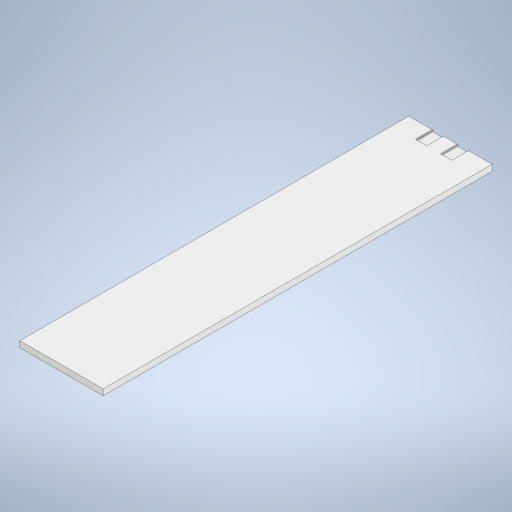
# Autodesk Inventor part: Resistance_chauffante_ceramique
Saved by Autodesk Inventor 2024 (Build 280153000, 153)
## iProperties
Created: 2024-08-30
Part Number: Resistance_chauffante_ceramique
Material: Générique
Document SubType Name: Modeling
Designer: malam
Density: 1 g/cm^3
Appearance: Par défaut
Author: malam
Autodesk Inventor part; units mm, degrees
ref_plane "YZ Plane" through (0, 0, 0) normal (1, 0, 0) x (0, 1, 0)
ref_plane "XZ Plane" through (0, 0, 0) normal (0, 1, 0) x (-1, 0, 0)
ref_plane "XY Plane" through (0, 0, 0) normal (0, 0, 1) x (1, 0, 0)
sketch "Esquisse1" plane through (0, 0, 0) normal (0, 1, 0) x (-1, 0, 0)
  line L0 (-7.5, 35) -> (7.5, 35)
  line L1 (7.5, 35) -> (7.5, -35)
  line L2 (7.5, -35) -> (-7.5, -35)
  line L3 (-7.5, -35) -> (-7.5, 35)
  line L4 (-7.5, 35) -> (7.5, -35) construction
  line L5 (7.5, 35) -> (-7.5, -35) construction
  point P0 (0, 0)
  dimension "d0" = 15
  dimension "d1" = 70
  constraints: 12 end point, 2 midpoint, 2 parallel, 1 horizontal, 1 perpendicular
  measures "d0" distance of L1.end L2.end
  measures "d1" distance of L0.end L1.end
extrude "Extrusion1" add sketch "Esquisse1" along normal blind 1.1
sketch "Esquisse2" plane through (0, 1.1, 0) normal (0, 1, 0) x (1, 0, 0)
  line L0 (7.5, 35) -> (-7.5, 35) projected
  line L1 (1.25, 35) -> (3.25, 35)
  line L2 (3.25, 35) -> (3.25, 32)
  line L3 (3.25, 32) -> (1.25, 32)
  line L4 (1.25, 32) -> (1.25, 35)
  line L5 (-3.25, 35) -> (-1.25, 35)
  line L6 (-1.25, 35) -> (-1.25, 32)
  line L7 (-1.25, 32) -> (-3.25, 32)
  line L8 (-3.25, 32) -> (-3.25, 35)
  line L9 (0, 35) -> (0, 28.8087) construction
  point P0 (0, 0)
  point P1 (-1.25, 33.5)
  dimension "d4" = 2
  dimension "d5" = 3
  dimension "d6" = 2
  dimension "d7" = 2.5
  dimension "d8" = 1.25
  constraints: 18 end point, 4 parallel, 3 point on line, 2 horizontal, 2 midpoint, 2 perpendicular, 1 vertical
  measures "d4" distance of L2.end L3.end
  measures "d5" distance of L1.end L2.end
  measures "d6" distance of L6.end L7.end
  measures "d7" distance between parallel lines of L4 L6
  measures "d8" distance from line of point (-1.25, 33.5) L9
extrude "Extrusion2" cut sketch "Esquisse2" against normal blind 0.3
